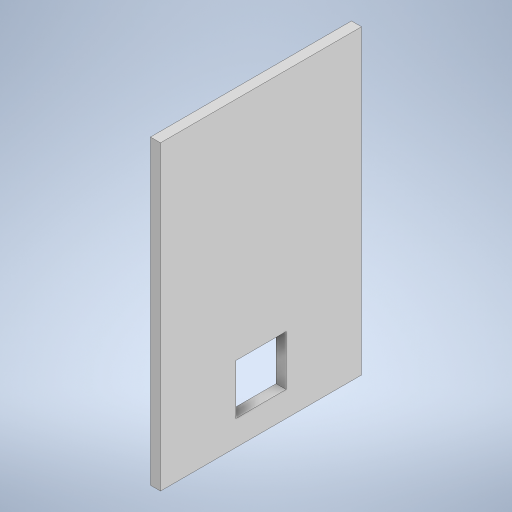
# Autodesk Inventor part: Left wall
Saved by Autodesk Inventor 2024.3 (Build 283343010, 343A)
## iProperties
Created: 2025-04-09
Part Number: Left wall
Material: Generic
Document SubType Name: Modeling
Designer: Vincent Larson
Density: 1 g/cm^3
Appearance: Default
Author: Vincent Larson
Autodesk Inventor part; units mm, degrees
ref_plane "YZ Plane" through (0, 0, 0) normal (1, 0, 0) x (0, 1, 0)
ref_plane "XZ Plane" through (0, 0, 0) normal (0, 1, 0) x (-1, 0, 0)
ref_plane "XY Plane" through (0, 0, 0) normal (0, 0, 1) x (1, 0, 0)
sketch "Sketch2" plane through (0, 0, 0) normal (1, 0, 0) x (0, 1, 0)
  line L0 (0, 0) -> (-152.4, 0)
  line L1 (-152.4, 0) -> (-152.4, -101.6)
  line L2 (-152.4, -101.6) -> (0, -101.6)
  line L3 (0, -101.6) -> (0, 0)
  dimension "d4" = 152.4
  dimension "d5" = 101.6
  constraints: 8 end point, 2 parallel, 1 horizontal, 1 perpendicular
  measures "d4" distance of L2.end L1.end
  measures "d5" distance of L1.end L0.end
extrude "Extrusion2" add sketch "Sketch2" along normal blind 5.08
sketch "Sketch4" plane through (5.08, 0, 0) normal (1, 0, 0) x (0, 0, -1)
  line L0 (0, -152.4) -> (101.6, -152.4) projected
  line L1 (50.8, -139.7) -> (63.5, -139.7)
  line L2 (63.5, -139.7) -> (38.1, -139.7)
  line L3 (38.1, -139.7) -> (38.1, -114.3)
  line L4 (38.1, -114.3) -> (63.5, -114.3)
  line L5 (63.5, -114.3) -> (63.5, -139.7)
  point P0 (0, 0)
  dimension "d13" = 12.7
  dimension "d14" = 25.4
  dimension "d15" = 25.4
  constraints: 10 end point, 2 parallel, 1 horizontal, 1 perpendicular
  measures "d13" distance of L1.start L1.end
  measures "d14" distance of L3.end L4.end
  measures "d15" distance of L2.end L3.end
extrude "Extrusion4" cut sketch "Sketch4" against normal blind 25.4
body "Solid2"
